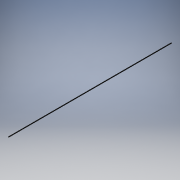
# Autodesk Inventor part: Hinge pin
Saved by Autodesk Inventor 2017 (Build 210142000, 142)
## iProperties
Shininess: 41.0
Length Units: 11272
Angle Units: 11279
Time Units: 11290
Mass Units: 11286
Length Display Precision: 3
Angle Display Precision: 2
Compacted: True
Created: 2001-09-30
Part Number: Hinge pin
Document SubType Name: Modeling
Designer: Tom Cross
Material: Generic
Density: 1 g/cm^3
Appearance: Glossy - Black
Density: 0.0
Volumn: 0.0
Area: 0.0
PropertySet Name: Model Information
Control State: 0
Master: False
Checked Out: False
Author: Tom Cross
Autodesk Inventor part; units mm, degrees
ref_plane "YZ Plane" through (0, 0, 0) normal (1, 0, 0) x (0, 1, 0)
ref_plane "XZ Plane" through (0, 0, 0) normal (0, 1, 0) x (-1, 0, 0)
ref_plane "XY Plane" through (0, 0, 0) normal (0, 0, 1) x (1, 0, 0)
sketch "Sketch1" plane through (0, 0, 0) normal (0, 0, 1) x (1, 0, 0)
  arc A0 (-3.048, 1.524) -> (-4.5488, 2.7834) centre (-3.048, 3.048) ccw projected
  circle A1 centre (-3.048, 3.048) radius 1.524
  constraints: 1 centre point, 1 coincident, 1 concentric
extrude "Extrusion1" add sketch "Sketch1" against normal blind 609.6
body "Solid1"
